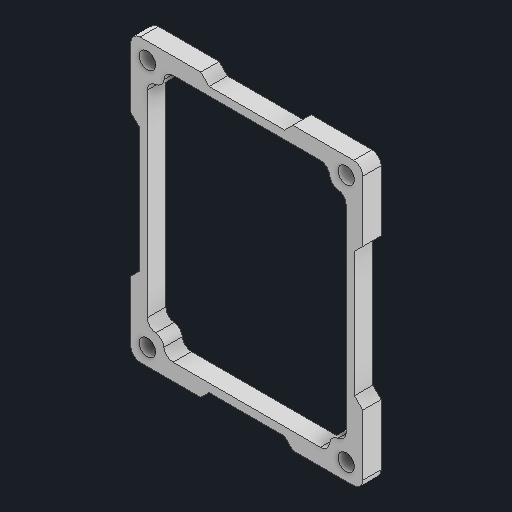
# Autodesk Inventor part: Servo-Gear-MountingPlate
Saved by Autodesk Inventor 2025 (Build 290162000, 162)
## iProperties
Created: 2024-05-18
Part Number: Servo-Gear-MountingPlate
Material: Generic
Document SubType Name: Modeling
Designer: zulet
Density: 1 g/cm^3
Appearance: Default
Author: zulet
Autodesk Inventor part; units mm, degrees
ref_plane "YZ Plane" through (0, 0, 0) normal (1, 0, 0) x (0, 1, 0)
ref_plane "XZ Plane" through (0, 0, 0) normal (0, 1, 0) x (-1, 0, 0)
ref_plane "XY Plane" through (0, 0, 0) normal (0, 0, 1) x (1, 0, 0)
sketch "Sketch1" plane through (0, 0, 0) normal (0, 0, 1) x (1, 0, 0)
  line L0 (0, 18) -> (0, 0) projected
  line L1 (0, 0) -> (18, 0) projected
  line L2 (18, 0) -> (18, 18) projected
  line L3 (18, 18) -> (0, 18) projected
  circle A0 centre (9, 9) radius 4.5 projected
  line L4 (0, 153) -> (18, 153) projected
  line L5 (0, 135) -> (0, 153) projected
  line L6 (18, 135) -> (0, 135) projected
  line L7 (18, 153) -> (18, 135) projected
  line L8 (0, 153) -> (18, 153) projected
  circle A1 centre (9, 144) radius 4.5 projected
  line L9 (126, 135) -> (126, 153) projected
  line L10 (126, 153) -> (108, 153) projected
  line L11 (108, 153) -> (108, 135) projected
  line L12 (108, 135) -> (126, 135) projected
  circle A2 centre (117, 144) radius 4.5 projected
  line L13 (126, 18) -> (126, 0) projected
  line L14 (108, 18) -> (126, 18) projected
  line L15 (108, 0) -> (108, 18) projected
  line L16 (126, 0) -> (108, 0) projected
  circle A3 centre (117, 9) radius 4.5 projected
  line L17 (18, 0) -> (108, 0)
  line L18 (108, 0) -> (108, 9)
  line L19 (108, 9) -> (18, 9)
  line L20 (18, 9) -> (18, 0)
  line L21 (126, 18) -> (117, 18)
  line L22 (117, 18) -> (117, 135)
  line L23 (117, 135) -> (126, 135)
  line L24 (126, 135) -> (126, 18)
  line L25 (108, 153) -> (18, 153)
  line L26 (18, 153) -> (18, 144)
  line L27 (18, 144) -> (108, 144)
  line L28 (108, 144) -> (108, 153)
  line L29 (0, 135) -> (9, 135)
  line L30 (9, 135) -> (9, 18)
  line L31 (9, 18) -> (0, 18)
  line L32 (0, 18) -> (0, 135)
  line L33 (126, 115) -> (121.5, 115)
  line L34 (121.5, 115) -> (121.5, 38)
  line L35 (121.5, 38) -> (126, 38)
  line L36 (126, 38) -> (126, 115)
  line L37 (88, 0) -> (38, 0)
  line L38 (38, 0) -> (38, 4.5)
  line L39 (38, 4.5) -> (88, 4.5)
  line L40 (88, 4.5) -> (88, 0)
  line L41 (0, 38) -> (4.5, 38)
  line L42 (4.5, 38) -> (4.5, 115)
  line L43 (4.5, 115) -> (0, 115)
  line L44 (0, 115) -> (0, 38)
  line L45 (38, 153) -> (88, 153)
  line L46 (88, 153) -> (88, 148.5)
  line L47 (88, 148.5) -> (38, 148.5)
  line L48 (38, 148.5) -> (38, 153)
  point P0 (18, 9)
  point P1 (38, 0)
  dimension "d0" = 9
  dimension "d1" = 9
  dimension "d2" = 9
  dimension "d3" = 9
  dimension "d4" = 4.5
  dimension "d5" = 4.5
  dimension "d6" = 4.5
  dimension "d7" = 4.5
  dimension "d8" = 20
  dimension "d9" = 20
  dimension "d10" = 20
  dimension "d11" = 20
  dimension "d12" = 20
  dimension "d13" = 20
  dimension "d14" = 20
  dimension "d15" = 20
  constraints: 64 end point, 16 parallel, 8 horizontal, 8 perpendicular, 4 midpoint, 4 point on line
  measures "d0" distance between parallel lines of L25 L27
  measures "d1" distance between parallel lines of L30 L32
  measures "d2" distance between parallel lines of L17 L19
  measures "d3" distance between parallel lines of L24 L22
  measures "d4" distance between parallel lines of L45 L47
  measures "d5" distance between parallel lines of L36 L34
  measures "d6" distance between parallel lines of L17 L39
  measures "d7" distance between parallel lines of L44 L42
  measures "d8" distance between parallel lines of L12 L33
  measures "d9" distance between parallel lines of L14 L35
  measures "d10" distance between parallel lines of L18 L40
  measures "d11" distance between parallel lines of L2 L38
  measures "d12" distance between parallel lines of L3 L41
  measures "d13" distance between parallel lines of L6 L43
  measures "d14" distance between parallel lines of L7 L48
  measures "d15" distance between parallel lines of L11 L46
extrude "Extrusion1" add sketch "Sketch1" along normal blind 10 contours L3 L2 L1 L0 | L32 L41 L42 L43 L6 L30 L3 | L2 L19 L15 L17 L40 L39 L38 | L6 L5 L4 L7 | L15 L14 L13 L16 | L7 L25 L48 L47 L46 L11 L27 | L11 L10 L9 L12 | L22 L12 L24 L33 L34 L35 L14
fillet "Fillet1" radius 5 16 edges at (108, 144, 5) (117, 135, 5) (108, 135, 5) (18, 144, 5) (18, 135, 5) (9, 135, 5) (9, 18, 5) (18, 18, 5) (18, 9, 5) (108, 9, 5) (108, 18, 5) (117, 18, 5) (0, 153, 5) (126, 153, 5) (126, 0, 5) (0, 0, 5)
chamfer "Chamfer1" distance 4.5 angle 45 8 edges at (38, 148.5, 5) (88, 148.5, 5) (121.5, 115, 5) (121.5, 38, 5) (38, 4.5, 5) (88, 4.5, 5) (4.5, 38, 5) (4.5, 115, 5)
equation "\"d1\" = d0"
equation "\"d2\" = d0"
equation "\"d3\" = d0"
equation "\"d4\" = 0.5 * d0"
equation "\"d5\" = 0.5 * d0"
equation "\"d6\" = 0.5 * d0"
equation "\"d7\" = 0.5 * d0"
equation "\"d9\" = d8"
equation "\"d10\" = d8"
equation "\"d11\" = d8"
equation "\"d12\" = d8"
equation "\"d13\" = d8"
equation "\"d14\" = d8"
equation "\"d15\" = d8"
body "Solid1"
